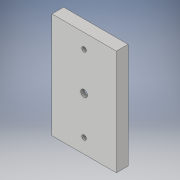
# Autodesk Inventor part: LightSwitchCover
Saved by Autodesk Inventor 2018 (Build 220112000, 112)
## iProperties
Created: 2018-02-16
Part Number: LightSwitchCover
Material: Generic
Document SubType Name: Modeling
Designer: brutu
Density: 1 g/cm^3
Appearance: Default
Author: brutu
Autodesk Inventor part; units mm, degrees
ref_plane "YZ Plane" through (0, 0, 0) normal (1, 0, 0) x (0, 1, 0)
ref_plane "XZ Plane" through (0, 0, 0) normal (0, 1, 0) x (-1, 0, 0)
ref_plane "XY Plane" through (0, 0, 0) normal (0, 0, 1) x (1, 0, 0)
sketch "Sketch1" plane through (0, 0, 0) normal (0, 0, 1) x (1, 0, 0)
  line L0 (0, 0) -> (69.85, 0)
  line L1 (69.85, 0) -> (69.85, 114.3)
  line L2 (69.85, 114.3) -> (0, 114.3)
  line L3 (0, 114.3) -> (0, 0)
  circle A0 centre (34.925, 98.552) radius 2.5
  circle A1 centre (34.925, 15.748) radius 2.5
  circle A2 centre (34.925, 57.15) radius 3.75
  point P0 (34.925, 114.3)
  point P1 (0, 57.15)
  dimension "d0" = 69.85
  dimension "d1" = 114.3
  dimension "d13" = 82.804
  dimension "d14" = 5
  dimension "d15" = 5
  dimension "d16" = 7.5
  dimension "d17" = 15.748
  constraints: 8 end point, 3 centre point, 3 vertical alignment, 2 midpoint, 2 parallel, 1 horizontal, 1 horizontal alignment, 1 perpendicular
  measures "d0" distance of L2.end L1.end
  measures "d1" distance of L1.end L0.end
  measures "d13" distance of A1.centre A0.centre
  measures "d14" diameter of A0
  measures "d15" diameter of A1
  measures "d16" diameter of A2
  measures "d17" distance from line of L2 A0.centre
extrude "Extrusion2" add sketch "Sketch1" along normal blind 12.7
sketch "Sketch3" plane through (0, 0, 0) normal (0, 0, -1) x (-1, 0, 0)
  line L0 (-66.04, 110.49) -> (-3.81, 110.49)
  line L1 (-3.81, 110.49) -> (-3.81, 3.81)
  line L2 (-3.81, 3.81) -> (-66.04, 3.81)
  line L3 (-66.04, 3.81) -> (-66.04, 110.49)
  circle A0 centre (-34.925, 57.15) radius 3.75 projected
  circle A1 centre (-34.925, 15.748) radius 2.5 projected
  circle A2 centre (-34.925, 98.552) radius 2.5 projected
  line L4 (0, 0) -> (-69.85, 0) projected
  line L5 (0, 114.3) -> (0, 0) projected
  line L6 (-69.85, 114.3) -> (0, 114.3) projected
  line L7 (-69.85, 0) -> (-69.85, 114.3) projected
  dimension "d20" = 114.3
  dimension "d21" = 69.85
  dimension "d22" = 3.81
  dimension "d24" = 3.81
  dimension "d25" = 3.81
  dimension "d26" = 3.81
  constraints: 8 end point, 2 parallel, 1 horizontal, 1 perpendicular
  measures "d20" distance of L4.end L6.start
  measures "d21" distance of L6.start L5.start
  measures "d22" distance between parallel lines of L3 L7
  measures "d24" distance between parallel lines of L6 L0
  measures "d25" distance between parallel lines of L1 L5
  measures "d26" distance between parallel lines of L4 L2
extrude "Extrusion3" cut sketch "Sketch3" against normal blind 8.89 contours L0 L1 L2 L3
sketch "Sketch4" plane through (0, 0, 8.89) normal (0, 0, -1) x (-1, 0, 0)
  circle A0 centre (-34.925, 57.15) radius 3.75 projected
  circle A1 centre (-34.925, 98.552) radius 2.5 projected
  circle A2 centre (-34.925, 15.748) radius 2.5 projected
  line L0 (-66.04, 110.49) -> (-3.81, 110.49) projected
  line L1 (-66.04, 3.81) -> (-66.04, 110.49) projected
  line L2 (-3.81, 3.81) -> (-66.04, 3.81) projected
  line L3 (-3.81, 110.49) -> (-3.81, 3.81) projected
  circle A3 centre (-58.42, 102.87) radius 3.175
  circle A4 centre (-58.42, 102.87) radius 1.25
  circle A5 centre (-11.43, 102.87) radius 3.175
  circle A6 centre (-11.43, 102.87) radius 1.25
  circle A7 centre (-58.42, 11.43) radius 3.175
  circle A8 centre (-58.42, 11.43) radius 1.25
  circle A9 centre (-11.43, 11.43) radius 3.175
  circle A10 centre (-11.43, 11.43) radius 1.25
  point P0 (0, 0)
  dimension "d29" = 6.35
  dimension "d30" = 2.5
  dimension "d31" = 6.35
  dimension "d32" = 2.5
  dimension "d33" = 7.62
  dimension "d34" = 7.62
  dimension "d35" = 7.62
  dimension "d36" = 7.62
  dimension "d37" = 6.35
  dimension "d38" = 2.5
  dimension "d39" = 7.62
  dimension "d40" = 7.62
  dimension "d41" = 6.35
  dimension "d42" = 2.5
  dimension "d43" = 7.62
  dimension "d44" = 7.62
  constraints: 8 centre point, 4 coincident
  measures "d29" diameter of A3
  measures "d30" diameter of A4
  measures "d31" diameter of A5
  measures "d32" diameter of A6
  measures "d33" distance from line of L0 A3.centre
  measures "d34" distance from line of L1 A3.centre
  measures "d35" distance from line of L0 A5.centre
  measures "d36" distance from line of L3 A5.centre
  measures "d37" diameter of A7
  measures "d38" diameter of A8
  measures "d39" distance from line of L1 A7.centre
  measures "d40" distance from line of L2 A7.centre
  measures "d41" diameter of A9
  measures "d42" diameter of A10
  measures "d43" distance from line of L3 A9.centre
  measures "d44" distance from line of L2 A9.centre
extrude "Extrusion4" add sketch "Sketch4" along normal blind 6.6 contours A3 | A5 | A7 | A9
equation "\"d17\" = -0.5 * d13 + 0.5 * d1"
equation "\"d24\" = d22"
equation "\"d25\" = d22"
equation "\"d26\" = d22"
equation "\"d31\" = d29"
equation "\"d32\" = d30"
equation "\"d34\" = d33"
equation "\"d35\" = d33"
equation "\"d36\" = d33"
equation "\"d37\" = d29"
equation "\"d38\" = d30"
equation "\"d39\" = d33"
equation "\"d40\" = d33"
equation "\"d41\" = d29"
equation "\"d42\" = d30"
equation "\"d43\" = d33"
equation "\"d44\" = d33"
body "Solid2"
